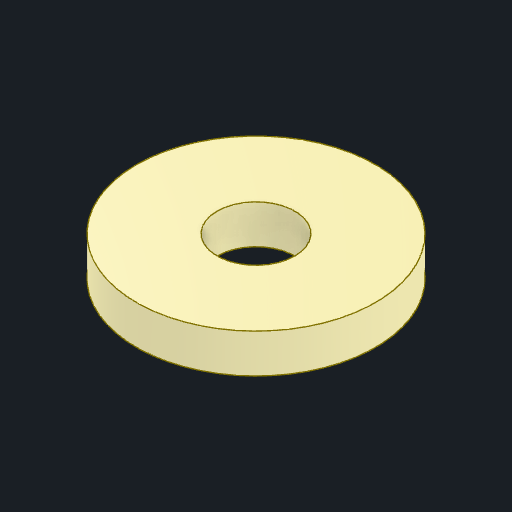
# Autodesk Inventor part: piniongear_41_middle
Saved by Autodesk Inventor 2022 (Build 260153000, 153)
## iProperties
Created: 2021-10-04
Part Number: piniongear_41_middle
Material: ナイロン 6/6
Document SubType Name: Modeling
Designer: shiok
Density: 1.13 g/cm^3
Appearance: ナイロン 6
Mass: 0.24014 g
Surface Area: 3.14929 cm^2
Volume: 0.212513 cm^3
Author: shiok
Autodesk Inventor part; units mm, degrees
ref_plane "YZ Plane" through (0, 0, 0) normal (1, 0, 0) x (0, 1, 0)
ref_plane "XZ Plane" through (0, 0, 0) normal (0, 1, 0) x (-1, 0, 0)
ref_plane "XY Plane" through (0, 0, 0) normal (0, 0, 1) x (1, 0, 0)
sketch "スケッチ1" plane through (0, 0, 0) normal (0, 1, 0) x (-1, 0, 0)
  circle A0 centre (0, 0) radius 6.15
  dimension "d0" = 12.3
  constraints: 1 centre point, 1 coincident
  measures "d0" diameter of A0
extrude "押し出し1" add sketch "スケッチ1" along normal blind 2
sketch "スケッチ2" plane through (0, 2, 0) normal (0, 1, 0) x (1, 0, 0)
  point P0 (0, 0)
  point P1 (0, 0)
  constraints: 1 coincident
hole "穴1" at (0, 2, 0) direction (0, -1, 0) diameter 4 end through all
